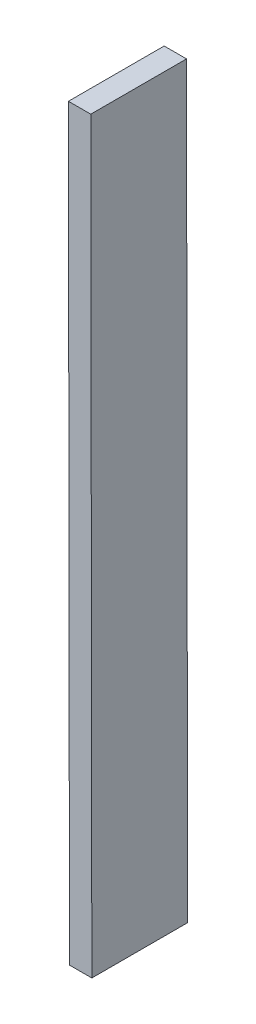
# Autodesk Inventor part: gira
Saved by Autodesk Inventor 2020 (Build 240168000, 168)
## iProperties
Created: 2022-10-31
Part Number: gira
Material: Generic
Document SubType Name: Modeling
Designer: super
Density: 1 g/cm^3
Appearance: Default
Author: super
Autodesk Inventor part; units mm, degrees
ref_plane "YZ Plane" through (0, 0, 0) normal (1, 0, 0) x (0, 1, 0)
ref_plane "XZ Plane" through (0, 0, 0) normal (0, 1, 0) x (-1, 0, 0)
ref_plane "XY Plane" through (0, 0, 0) normal (0, 0, 1) x (1, 0, 0)
ref_plane "Work Plane1" through (-84.5679, -177.7614, 10.4079) normal (0.999999, 0.0014131, 0) x (0.0014131, -0.999999, 0)
sketch "Sketch1" plane through (-84.5679, -177.7614, 10.4079) normal (0.999999, 0.0014131, 0) x (0.0014131, -0.999999, 0)
  line L0 (9.6295, -13.989) -> (-157.4911, -13.989)
  line L1 (-157.4911, -13.989) -> (-157.4911, 7.4134)
  line L2 (-157.4911, 7.4134) -> (9.6295, 7.4134)
  line L3 (9.6295, 7.4134) -> (9.6295, -13.989)
  point P0 (-177.6417, 10.4079)
  constraints: 8 end point, 2 parallel, 1 horizontal, 1 perpendicular
extrude "Extrusion1" add sketch "Sketch1" along normal blind 5
body "Solid1"
